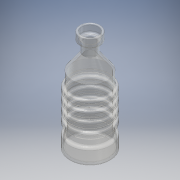
# Autodesk Inventor part: botella
Saved by Autodesk Inventor 2016 (Build 200138000, 138)
## iProperties
Created: 2016-09-16
Part Number: botella
Material: Plástico, transparente
Document SubType Name: Modeling
Designer: Isabel
Density: 1.188 g/cm^3
Appearance: Transparente - Claro
Author: Isabel
Autodesk Inventor part; units mm, degrees
ref_plane "YZ Plane" through (0, 0, 0) normal (1, 0, 0) x (0, 1, 0)
ref_plane "XZ Plane" through (0, 0, 0) normal (0, 1, 0) x (-1, 0, 0)
ref_plane "XY Plane" through (0, 0, 0) normal (0, 0, 1) x (1, 0, 0)
sketch "Boceto1" plane through (0, 0, 0) normal (0, 0, 1) x (1, 0, 0)
  line L0 (0, 0) -> (37, 0)
  line L1 (40, 3) -> (40, 27)
  line L2 (37, 30) -> (37.8316, 30)
  line L3 (34.8316, 33) -> (34.8316, 41)
  line L4 (37.8316, 44) -> (37, 44)
  line L5 (40, 47) -> (40, 53)
  line L6 (37, 56) -> (37.8316, 56)
  line L7 (34.8316, 59) -> (34.8316, 59)
  line L8 (37.8316, 62) -> (37, 62)
  line L9 (40, 65) -> (40, 71)
  line L10 (37, 74) -> (37.8316, 74)
  line L11 (34.8316, 77) -> (34.8316, 77)
  line L12 (37.8316, 80) -> (37, 80)
  line L13 (40, 83) -> (40, 89)
  line L14 (37, 92) -> (37.8316, 92)
  line L15 (34.8316, 95) -> (34.8316, 95.029)
  line L16 (37.8316, 98.029) -> (37, 98.029)
  line L17 (40, 101.029) -> (40, 107.029)
  line L18 (37, 110.029) -> (37.8316, 110.029)
  line L19 (34.8316, 113.029) -> (34.8316, 135.029)
  line L20 (34.8316, 135.029) -> (13, 165.029)
  line L21 (13, 165.029) -> (13, 181)
  line L22 (16, 184) -> (17, 184)
  line L23 (20, 187) -> (20, 200)
  arc A0 (34.8316, 113.029) -> (37.8316, 110.029) centre (37.8316, 113.029) ccw
  arc A1 (40, 107.029) -> (37, 110.029) centre (37, 107.029) ccw
  arc A2 (37, 98.029) -> (40, 101.029) centre (37, 101.029) ccw
  arc A3 (37.8316, 98.029) -> (34.8316, 95.029) centre (37.8316, 95.029) ccw
  arc A4 (34.8316, 95) -> (37.8316, 92) centre (37.8316, 95) ccw
  arc A5 (40, 89) -> (37, 92) centre (37, 89) ccw
  arc A6 (37, 80) -> (40, 83) centre (37, 83) ccw
  arc A7 (37.8316, 80) -> (34.8316, 77) centre (37.8316, 77) ccw
  arc A8 (34.8316, 77) -> (37.8316, 74) centre (37.8316, 77) ccw
  arc A9 (40, 71) -> (37, 74) centre (37, 71) ccw
  arc A10 (37, 62) -> (40, 65) centre (37, 65) ccw
  arc A11 (37.8316, 62) -> (34.8316, 59) centre (37.8316, 59) ccw
  arc A12 (34.8316, 59) -> (37.8316, 56) centre (37.8316, 59) ccw
  arc A13 (40, 53) -> (37, 56) centre (37, 53) ccw
  arc A14 (37, 44) -> (40, 47) centre (37, 47) ccw
  arc A15 (37.8316, 44) -> (34.8316, 41) centre (37.8316, 41) ccw
  arc A16 (34.8316, 33) -> (37.8316, 30) centre (37.8316, 33) ccw
  arc A17 (40, 27) -> (37, 30) centre (37, 27) ccw
  arc A18 (37, 0) -> (40, 3) centre (37, 3) ccw
  arc A19 (16, 184) -> (13, 181) centre (16, 181) ccw
  arc A20 (17, 184) -> (20, 187) centre (17, 187) ccw
  line L24 (16, 190) -> (16, 200)
  line L25 (13, 187) -> (10, 187)
  line L26 (10, 184) -> (10, 162.029)
  line L27 (10, 162.029) -> (31.8316, 132.029)
  line L28 (31.8316, 132.029) -> (31.8316, 110.029)
  line L29 (34.8316, 107.029) -> (34, 107.029)
  line L30 (37, 104.029) -> (37, 104.029)
  line L31 (34, 101.029) -> (34.8316, 101.029)
  line L32 (31.8316, 98.029) -> (31.8316, 92)
  line L33 (34.8316, 89) -> (37, 89)
  line L34 (37, 86.0579) -> (37, 86)
  line L35 (34, 83) -> (31.8316, 83)
  line L36 (31.8316, 80.0579) -> (31.8316, 74)
  line L37 (34.8316, 71) -> (34, 71)
  line L38 (37, 68) -> (37, 68)
  line L39 (34, 65) -> (34.8316, 65)
  line L40 (31.8316, 62) -> (31.8316, 56)
  line L41 (34.8316, 53) -> (34, 53)
  line L42 (37, 50) -> (37, 50)
  line L43 (34, 47) -> (34.8316, 47)
  line L44 (31.8316, 44) -> (31.8316, 30)
  line L45 (34.8316, 27) -> (34, 27)
  line L46 (37, 24) -> (37, 6)
  line L47 (34, 3) -> (0, 3)
  line L48 (0, 3) -> (0, 0)
  arc A21 (20, 200) -> (16, 200) centre (18, 200) ccw
  arc A22 (13, 187) -> (16, 190) centre (13, 190) ccw
  arc A23 (13, 187) -> (10, 184) centre (13, 184) ccw
  arc A24 (31.8316, 110.029) -> (34.8316, 107.029) centre (34.8316, 110.029) ccw
  arc A25 (37, 104.029) -> (34, 107.029) centre (34, 104.029) ccw
  arc A26 (34, 101.029) -> (37, 104.029) centre (34, 104.029) ccw
  arc A27 (34.8316, 101.029) -> (31.8316, 98.029) centre (34.8316, 98.029) ccw
  arc A28 (31.8316, 92) -> (34.4158, 89.029) centre (34.8316, 92) ccw
  arc A29 (37, 86.0579) -> (34.4158, 89.029) centre (34, 86.0579) ccw
  arc A30 (34.4158, 83.029) -> (37, 86) centre (34, 86) ccw
  arc A31 (34.4158, 83.029) -> (31.8316, 80.0579) centre (34.8316, 80.0579) ccw
  arc A32 (31.8316, 74) -> (34.8316, 71) centre (34.8316, 74) ccw
  arc A33 (37, 68) -> (34, 71) centre (34, 68) ccw
  arc A34 (34, 65) -> (37, 68) centre (34, 68) ccw
  arc A35 (34.8316, 65) -> (31.8316, 62) centre (34.8316, 62) ccw
  arc A36 (31.8316, 56) -> (34.8316, 53) centre (34.8316, 56) ccw
  arc A37 (37, 50) -> (34, 53) centre (34, 50) ccw
  arc A38 (34, 47) -> (37, 50) centre (34, 50) ccw
  arc A39 (34.8316, 47) -> (31.8316, 44) centre (34.8316, 44) ccw
  arc A40 (31.8316, 30) -> (34.8316, 27) centre (34.8316, 30) ccw
  arc A41 (37, 24) -> (34, 27) centre (34, 24) ccw
  arc A42 (34, 3) -> (37, 6) centre (34, 6) ccw
  point P0 (40, 0)
  point P1 (40, 30)
  point P2 (34.8316, 44)
  point P3 (40, 44)
  point P4 (40, 56)
  point P5 (34.8316, 62)
  point P6 (40, 62)
  point P7 (40, 74)
  point P8 (34.8316, 80)
  point P9 (40, 80)
  point P10 (40, 92)
  point P11 (34.8316, 92)
  point P12 (34.8316, 98.029)
  point P13 (40, 98.029)
  point P14 (40, 110.029)
  point P15 (34.8316, 110.029)
  point P16 (13, 184)
  point P17 (20, 200)
  point P18 (31.8316, 101.029)
  point P19 (31.8316, 89)
  point P20 (33.2074, 89)
  point P21 (37, 65)
  point P22 (31.8316, 65)
  point P23 (31.8316, 53)
  point P24 (37, 47)
  point P25 (31.8316, 47)
  point P26 (31.8316, 27)
  point P27 (37, 27)
  point P28 (37, 3)
  dimension "d1" = 30
  dimension "d2" = 25
  dimension "d5" = 12
  dimension "d7" = 12
  dimension "d9" = 12
  dimension "d13" = 40
  dimension "d14" = 3
  dimension "d15" = 3
  dimension "d16" = 3
  dimension "d17" = 3
  dimension "d18" = 3
  dimension "d19" = 3
  dimension "d20" = 3
  dimension "d21" = 3
  dimension "d22" = 3
  dimension "d23" = 3
  dimension "d24" = 3
  dimension "d25" = 3
  dimension "d26" = 3
  dimension "d27" = 3
  dimension "d28" = 3
  dimension "d29" = 3
  dimension "d30" = 3
  dimension "d31" = 3
  dimension "d32" = 3
  dimension "d34" = 3
  dimension "d37" = 3
  dimension "d38" = 3
  dimension "d39" = 3
  dimension "d40" = 3
  dimension "d43" = 3
  dimension "d44" = 3
  dimension "d45" = 3
  dimension "d46" = 3
  dimension "d47" = 3
  dimension "d48" = 3
  dimension "d49" = 3
  dimension "d50" = 3
  dimension "d51" = 3
  dimension "d52" = 3
  dimension "d53" = 3
  dimension "d54" = 3
  dimension "d55" = 2
  dimension "d56" = 3
  dimension "d57" = 3
  dimension "d58" = 3
  dimension "d59" = 3
  dimension "d61" = 12
  dimension "d62" = 12
  dimension "d63" = 20
  dimension "d64" = 12
  dimension "d65" = 12
  dimension "d66" = 200
  dimension "d67" = 3
  dimension "d68" = 3
  dimension "d70" = 30
  dimension "d73" = 10
  dimension "d74" = 25
  dimension "d75" = 20
  dimension "d76" = 16
  constraints: 98 end point, 96 point on line, 89 point on circle, 86 tangent, 43 centre point, 26 perpendicular, 16 equal radius, 3 horizontal, 3 parallel, 3 vertical, 1 horizontal alignment, 2 other
  measures "d1" distance of point (40, 30) point (40, 0)
  measures "d2" vertical distance of point (40, 110.029) L19.end
  measures "d5" distance of point (40, 80) point (40, 92)
  measures "d7" distance of point (40, 62) point (40, 74)
  measures "d9" vertical distance of point (40, 44) point (34.832, 56)
  measures "d13" distance of L0.start point (40, 0)
  measures "d14" radius of A0
  measures "d15" radius of A1
  measures "d16" radius of A2
  measures "d17" radius of A3
  measures "d18" radius of A4
  measures "d19" radius of A5
  measures "d20" radius of A6
  measures "d21" radius of A7
  measures "d22" radius of A8
  measures "d23" radius of A9
  measures "d24" radius of A10
  measures "d25" radius of A11
  measures "d26" radius of A12
  measures "d27" radius of A13
  measures "d28" radius of A14
  measures "d29" radius of A15
  measures "d30" radius of A16
  measures "d31" radius of A17
  measures "d32" radius of A18
  measures "d34" radius of A19
  measures "d37" distance between parallel lines of L0 L47
  measures "d38" distance between parallel lines of L1 L46
  measures "d39" distance between parallel lines of L44 L3
  measures "d40" distance from line of L45 L2.end
  measures "d43" distance of point (37, 53) L6.start
  measures "d44" distance from line of L8.start L39
  measures "d45" distance from line of L4.end L43
  measures "d46" distance from line of L10.start L37
  measures "d47" distance from line of L12.end L35
  measures "d48" distance from line of L14.start L33
  measures "d49" distance between parallel lines of L15 L32
  measures "d50" distance from line of L16.end L31
  measures "d51" distance from line of L29 L18.end
  measures "d52" distance between parallel lines of L17 L30
  measures "d53" distance between parallel lines of L26 L21
  measures "d54" distance from line of L25 L22.end
  measures "d55" radius of A21
  measures "d56" radius of A22
  measures "d57" radius of A23
  measures "d58" radius of A24
  measures "d59" radius of A28
  measures "d61" distance of L16.start L18.end
  measures "d62" vertical distance of A28.end L31.start
  measures "d63" distance between parallel lines of L43 L45
  measures "d64" distance between parallel lines of L39 L41
  measures "d65" vertical distance of L37.start L35.start
  measures "d66" distance from line of L0 A21.centre
  measures "d67" radius of A33
  measures "d68" radius of A42
  measures "d70" vertical distance of L19.end L20.end
  measures "d73" distance from line of L0.start L26
  measures "d74" vertical distance of L29.start L27.end
  measures "d75" distance from line of L47.end L23
  measures "d76" vertical distance of A21.centre L22.start
revolve "Revolución1" add sketch "Boceto1" angle 360 about axis through (0, 3, 0) along (0, -1, 0)
move or copy body "Desplazar cuerpo1" bodies to move or copy 1 copy no rotation origin (0, 0, 0) rotation axis (1, 0, 0) rotation angle 90
